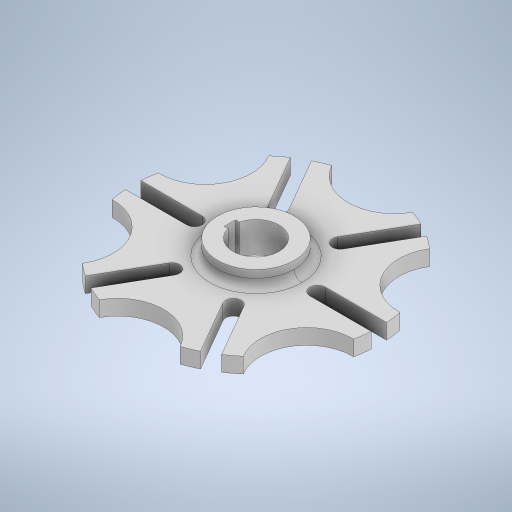
# Autodesk Inventor part: Pieza4-Tarea1
Saved by Autodesk Inventor 2024 (Build 280153000, 153)
## iProperties
Created: 2024-02-16
Part Number: Pieza4-Tarea1
Material: Genérico
Document SubType Name: Modeling
Designer: Diegolap
Density: 1 g/cm^3
Appearance: Valor por defecto
Mass: 279.199 g
Surface Area: 623.937 cm^2
Volume: 279.199 cm^3
Author: Diegolap
Autodesk Inventor part; units mm, degrees
ref_plane "YZ Plane" through (0, 0, 0) normal (1, 0, 0) x (0, 1, 0)
ref_plane "XZ Plane" through (0, 0, 0) normal (0, 1, 0) x (-1, 0, 0)
ref_plane "XY Plane" through (0, 0, 0) normal (0, 0, 1) x (1, 0, 0)
sketch "Boceto1" plane through (0, 0, 0) normal (0, 1, 0) x (-1, 0, 0)
  circle A0 centre (0, 0) radius 101.6
  line L0 (0, 0) -> (101.6, 0)
  line L1 (0, 0) -> (0, 50.8)
  line L2 (0, 0) -> (0, -50.8)
  line L3 (0, 0) -> (-101.6, 0)
  line L4 (0, 0) -> (50.8, -87.9882)
  line L5 (0, 0) -> (50.8, 87.9882)
  line L6 (0, 0) -> (-50.8, -87.9882)
  line L7 (0, 0) -> (-50.8, 87.9882)
  circle A1 centre (0, 0) radius 50.8
  line L8 (101.6, 0) -> (50.8, 0) construction
  line L9 (101.6, 6.35) -> (50.8, 6.35)
  line L10 (50.8, -6.35) -> (101.6, -6.35)
  arc A2 (101.6, -6.35) -> (101.6, 6.35) centre (101.6, 0) ccw
  arc A3 (50.8, 6.35) -> (50.8, -6.35) centre (50.8, 0) ccw
  line L11 (50.8, -87.9882) -> (25.4, -43.9941) construction
  line L12 (56.2993, -84.8132) -> (30.8993, -40.8191)
  line L13 (19.9007, -47.1691) -> (45.3007, -91.1632)
  arc A4 (45.3007, -91.1632) -> (56.2993, -84.8132) centre (50.8, -87.9882) ccw
  arc A5 (30.8993, -40.8191) -> (19.9007, -47.1691) centre (25.4, -43.9941) ccw
  line L14 (0, -57.15) -> (0, -50.8) construction
  line L15 (6.35, -101.6) -> (6.35, -101.4014)
  line L16 (-6.35, -101.4014) -> (-6.35, -101.6)
  line L17 (-50.8, -87.9882) -> (-25.4, -43.9941) construction
  line L18 (-45.3007, -91.1632) -> (-19.9007, -47.1691)
  line L19 (-30.8993, -40.8191) -> (-56.2993, -84.8132)
  arc A6 (-56.2993, -84.8132) -> (-45.3007, -91.1632) centre (-50.8, -87.9882) ccw
  arc A7 (-19.9007, -47.1691) -> (-30.8993, -40.8191) centre (-25.4, -43.9941) ccw
  line L20 (-101.6, 0) -> (-50.8, 0) construction
  line L21 (-101.6, -6.35) -> (-50.8, -6.35)
  line L22 (-50.8, 6.35) -> (-101.6, 6.35)
  arc A8 (-101.6, 6.35) -> (-101.6, -6.35) centre (-101.6, 0) ccw
  arc A9 (-50.8, -6.35) -> (-50.8, 6.35) centre (-50.8, 0) ccw
  line L23 (-50.8, 87.9882) -> (-25.4, 43.9941) construction
  line L24 (-45.3007, 91.1632) -> (-19.9007, 47.1691)
  line L25 (-30.8993, 40.8191) -> (-56.2993, 84.8132)
  arc A10 (-45.3007, 91.1632) -> (-56.2993, 84.8132) centre (-50.8, 87.9882) ccw
  arc A11 (-30.8993, 40.8191) -> (-19.9007, 47.1691) centre (-25.4, 43.9941) ccw
  line L26 (50.8, 87.9882) -> (25.4, 43.9941) construction
  line L27 (45.3007, 91.1632) -> (19.9007, 47.1691)
  line L28 (30.8993, 40.8191) -> (56.2993, 84.8132)
  arc A12 (56.2993, 84.8132) -> (45.3007, 91.1632) centre (50.8, 87.9882) ccw
  arc A13 (19.9007, 47.1691) -> (30.8993, 40.8191) centre (25.4, 43.9941) ccw
  line L29 (0, 101.6) -> (0, 50.8) construction
  line L30 (-6.35, 101.6) -> (-6.35, 101.4014)
  line L31 (6.35, 101.4014) -> (6.35, 101.6)
  circle A14 centre (0, 0) radius 114.3
  arc A15 (6.35, -50.8) -> (6.3376, -50.4031) centre (0, -50.8) ccw
  arc A16 (-6.3376, -50.4031) -> (-6.35, -50.8) centre (0, -50.8) ccw
  arc A17 (-6.35, 50.8) -> (-6.3376, 50.4031) centre (0, 50.8) ccw
  arc A18 (6.3376, 50.4031) -> (6.35, 50.8) centre (0, 50.8) ccw
  circle A19 centre (0, 114.3) radius 38.1
  circle A20 centre (0, -114.3) radius 38.1
  line L32 (0, 0) -> (98.9867, -57.15)
  circle A21 centre (98.9867, -57.15) radius 38.1
  line L33 (0, 0) -> (98.9867, 57.15)
  circle A22 centre (98.9867, 57.15) radius 38.1
  line L34 (0, 0) -> (-98.9867, 57.15)
  line L35 (0, 0) -> (-98.9867, -57.15)
  circle A23 centre (-98.9867, 57.15) radius 38.1
  circle A24 centre (-98.9867, -57.15) radius 38.1
  point P0 (76.2, 0)
  point P1 (38.1, -65.9911)
  point P2 (0, -76.2)
  point P3 (-38.1, -65.9911)
  point P4 (-76.2, 0)
  point P5 (-38.1, 65.9911)
  point P6 (38.1, 65.9911)
  point P7 (0, 76.2)
  point P8 (-56.1999, 84.6412)
  point P9 (-66.4035, 76.8969)
  point P10 (-99.7964, 19.0586)
  point P11 (-101.4014, 6.35)
  point P12 (-101.4014, -6.35)
  point P13 (-99.7964, -19.0586)
  point P14 (-66.4035, -76.8969)
  point P15 (-56.1999, -84.6412)
  point P16 (-45.2014, -90.9912)
  point P17 (-33.393, -95.9556)
  point P18 (33.393, -95.9556)
  point P19 (45.2014, -90.9912)
  point P20 (56.1999, -84.6412)
  point P21 (66.4035, -76.8969)
  point P22 (99.7964, -19.0586)
  point P23 (101.4014, -6.35)
  point P24 (101.4014, 6.35)
  point P25 (99.7964, 19.0586)
  point P26 (66.4035, 76.8969)
  point P27 (56.1999, 84.6412)
  point P28 (45.2014, 90.9912)
  point P29 (33.393, 95.9556)
  point P30 (-33.393, 95.9556)
  point P31 (-45.2014, 90.9912)
  dimension "d0" = 203.2
  dimension "d5" = 101.6
  dimension "d1" = 60
  dimension "d2" = 60
  dimension "d3" = 60
  dimension "d4" = 60
  dimension "d6" = 12.7
  dimension "d7" = 12.7
  dimension "d8" = 12.7
  dimension "d9" = 12.7
  dimension "d10" = 12.7
  dimension "d11" = 12.7
  dimension "d12" = 12.7
  dimension "d13" = 12.7
  dimension "d14" = 228.6
  dimension "d15" = 30
  dimension "d16" = 76.2
  dimension "d17" = 30
  dimension "d18" = 76.2
  dimension "d19" = 30
  dimension "d20" = 30
  dimension "d21" = 76.2
  dimension "d22" = 76.2
  constraints: 88 end point, 39 point on circle, 28 tangent, 21 centre point, 13 midpoint, 8 parallel, 7 coincident, 2 point on line, 1 horizontal, 1 perpendicular, 33 other
  measures "d1" angle of L0 L4
  measures "d2" angle of L0 L5
  measures "d3" angle of L3 L6
  measures "d4" angle of L3 L7
  measures "d6" distance between parallel lines of L9 L10
  measures "d7" distance between parallel lines of L12 L13
  measures "d8" distance between parallel lines of L16 L15
  measures "d9" distance between parallel lines of L19 L18
  measures "d10" distance between parallel lines of L22 L21
  measures "d11" distance between parallel lines of L24 L25
  measures "d12" distance between parallel lines of L31 L30
  measures "d13" distance between parallel lines of L28 L27
  measures "d14" diameter of A14
  measures "d15" angle of L0 L32
  measures "d16" diameter of A21
  measures "d17" angle of L33 L0
  measures "d18" diameter of A22
  measures "d19" angle of L3 L34
  measures "d20" angle of L3 L35
  measures "d21" diameter of A23
  measures "d22" diameter of A24
extrude "Extrusión1" add sketch "Boceto1" along normal blind 12.7 contours A0 L27 A13 A1 A11 L24 A19 | A0 A22 L33 A1 A13 L28 | A13 L5 L1 A1 | L25 A11 A1 L34 A23 A0 | A1 L1 L7 A11 | A13 A1 L33 L5 | A22 A0 L9 A3 A1 L33 | L7 L34 A1 A11 | A23 L34 A1 A9 L22 A0 | L33 A1 A3 L0 | L4 A5 A1 L2 | L35 A1 A9 L3 | L32 A1 A5 L4 | L2 A1 A7 L6 | L0 A3 A1 L32 | L3 A9 A1 L34 | L6 A7 A1 L35 | A0 L21 A9 A1 L35 A24 | A1 A5 L13 A0 A20 L18 A7 | L32 A21 A0 L12 A5 A1 | A1 A3 L10 A0 A21 L32 | A1 A7 L19 A0 A24 L35
sketch "Boceto2" plane through (0, 12.7, 0) normal (0, 1, 0) x (1, 0, 0)
  circle A0 centre (0, 0) radius 31.75
  dimension "d25" = 63.5
  constraints: 1 centre point, 1 coincident
  measures "d25" diameter of A0
extrude "Extrusión2" add sketch "Boceto2" along normal blind 12.7
sketch "Boceto3" plane through (0, 25.4, 0) normal (0, 1, 0) x (1, 0, 0)
  circle A0 centre (0, 0) radius 19.05
  dimension "d28" = 38.1
  constraints: 1 centre point, 1 coincident
  measures "d28" diameter of A0
sketch "Boceto4" plane through (0, 12.7, 0) normal (0, 1, 0) x (1, 0, 0)
  point P0 (0, 0)
fillet "Empalme1" radius 6.35 1 edges at (-31.75, 12.7, 0) curvature continuous yes
sketch "Boceto5" plane through (0, 25.4, 0) normal (0, 1, 0) x (1, 0, 0)
  line L0 (0, 0) -> (-31.75, 0)
  circle A0 centre (0, 0) radius 31.75 projected
  line L1 (-16.51, -4.572) -> (-21.59, -4.572)
  line L2 (-21.59, -4.572) -> (-21.59, 4.572)
  line L3 (-21.59, 4.572) -> (-16.51, 4.572)
  line L4 (-16.51, 4.572) -> (-16.51, -4.572)
  line L5 (-16.51, -4.572) -> (-21.59, 4.572) construction
  line L6 (-21.59, -4.572) -> (-16.51, 4.572) construction
  point P0 (-19.05, 0)
  dimension "d30" = 9.144
  dimension "d31" = 5.08
  dimension "d32" = 19.05
  constraints: 14 end point, 2 horizontal, 2 midpoint, 2 parallel, 1 horizontal alignment, 1 perpendicular, 1 point on line, 1 other
  measures "d30" distance of L1.end L2.end
  measures "d31" distance of L2.end L3.end
  measures "d32" distance of L0.start point (-19.05, 0)
extrude "Extrusión3" cut sketch "Boceto3" against normal blind 25.4
extrude "Extrusión4" cut sketch "Boceto5" against normal blind 25.4 contours L4 L1 L2 L0 | L0 L2 L3 L4
